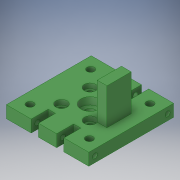
# Autodesk Inventor part: КВ33.044.201 - Щека каретки
Saved by Autodesk Inventor 2019 (Build 230136000, 136)
## iProperties
Created: 2019-07-18
Part Number: КВ33.044.201 - Щека каретки
Material: Пластик АБС
Document SubType Name: Modeling
Designer: Петров Иван
Density: 1.06 g/cm^3
Appearance: Гладкий — темный травянисто-зеленый
Author: Петров Иван
Autodesk Inventor part; units mm, degrees
ref_plane "YZ Plane" through (0, 0, 0) normal (1, 0, 0) x (0, 1, 0)
ref_plane "XZ Plane" through (0, 0, 0) normal (0, 1, 0) x (-1, 0, 0)
ref_plane "XY Plane" through (0, 0, 0) normal (0, 0, 1) x (1, 0, 0)
sketch "Эскиз1" plane through (0, 0, 0) normal (0, 1, 0) x (-1, 0, 0)
  line L0 (-34, 35) -> (34, 35)
  line L1 (34, 35) -> (34, -35)
  line L2 (34, -35) -> (-34, -35)
  line L3 (-34, -35) -> (-34, 35)
  line L4 (-34, 35) -> (34, -35) construction
  line L5 (34, 35) -> (-34, -35) construction
  line L6 (0, -35) -> (0, -25)
  line L7 (0, -25) -> (24.48, -25)
  line L8 (0, -25) -> (-24.48, -25)
  circle A0 centre (24.48, -25) radius 3
  circle A1 centre (-24.48, -25) radius 3
  line L9 (0, 35) -> (0, 25)
  line L10 (0, 25) -> (24.48, 25)
  line L11 (0, 25) -> (24.48, 25) construction
  line L12 (0, 25) -> (-24.48, 25)
  circle A2 centre (-24.48, 25) radius 3
  circle A3 centre (24.48, 25) radius 3
  arc A4 (3.9646, 5.9999) -> (5.0253, 6.4392) centre (3.9646, 7.4999) ccw
  line L13 (3.9646, 5.9999) -> (0.7747, 5.9999)
  line L14 (0.7747, 5.9999) -> (0.0002, 5.35)
  line L15 (0.0002, 5.35) -> (-0.7746, 6.0001)
  line L16 (-0.7746, 6.0001) -> (-3.9642, 6.0001)
  arc A5 (-5.0249, 6.4394) -> (-3.9642, 6.0001) centre (-3.9642, 7.5001) ccw
  line L17 (-5.0249, 6.4394) -> (-8.3536, 9.7681)
  arc A6 (-8.5, 10.1217) -> (-8.3536, 9.7681) centre (-8, 10.1217) ccw
  line L18 (-8.5, 10.1217) -> (-8.5, 12.6)
  arc A7 (-8.3, 12.8) -> (-8.5, 12.6) centre (-8.3, 12.6) ccw
  line L19 (-8.3, 12.8) -> (-4.3, 12.8)
  arc A8 (-4.3, 12.8) -> (-4.1, 13) centre (-4.3, 13) ccw
  line L20 (-4.1, 13) -> (-4.1, 14.1)
  arc A9 (-4.1, 14.1) -> (-4.3, 14.3) centre (-4.3, 14.1) ccw
  line L21 (-4.3, 14.3) -> (-4.7, 14.3)
  line L22 (-4.7, 14.3) -> (-4.7, 14.8001)
  arc A10 (-4.7, 14.8001) -> (-4.9001, 15.0001) centre (-4.9001, 14.8001) ccw
  line L23 (-4.9001, 15.0001) -> (-13.5, 15.0001)
  arc A11 (-13.5, 15.0001) -> (-15, 13.5001) centre (-13.5, 13.5001) ccw
  line L24 (-15, 13.5001) -> (-15, 4.8999)
  arc A12 (-15, 4.8999) -> (-14.8, 4.6999) centre (-14.8, 4.8999) ccw
  line L25 (-14.8, 4.6999) -> (-14.3, 4.6999)
  line L26 (-14.3, 4.6999) -> (-14.3, 4.2999)
  arc A13 (-14.3, 4.2999) -> (-14.1, 4.0999) centre (-14.1, 4.2999) ccw
  line L27 (-14.1, 4.0999) -> (-13, 4.0999)
  arc A14 (-13, 4.0999) -> (-12.8, 4.2999) centre (-13, 4.2999) ccw
  line L28 (-12.8, 4.2999) -> (-12.8, 8.3)
  arc A15 (-12.6, 8.5) -> (-12.8, 8.3) centre (-12.6, 8.3) ccw
  line L29 (-12.6, 8.5) -> (-10.1211, 8.5)
  arc A16 (-9.7675, 8.3536) -> (-10.1211, 8.5) centre (-10.1211, 8) ccw
  line L30 (-9.7675, 8.3536) -> (-6.4392, 5.0253)
  arc A17 (-5.9999, 3.9646) -> (-6.4392, 5.0253) centre (-7.4999, 3.9646) ccw
  line L31 (-5.9999, 3.9646) -> (-5.9999, 0.7747)
  line L32 (-5.9999, 0.7747) -> (-5.35, 0.0002)
  line L33 (-5.35, 0.0002) -> (-6.0001, -0.7746)
  line L34 (-6.0001, -0.7746) -> (-6.0001, -3.9642)
  arc A18 (-6.4394, -5.0249) -> (-6.0001, -3.9642) centre (-7.5001, -3.9642) ccw
  line L35 (-6.4394, -5.0249) -> (-9.7681, -8.3536)
  arc A19 (-10.1217, -8.5) -> (-9.7681, -8.3536) centre (-10.1217, -8) ccw
  line L36 (-10.1217, -8.5) -> (-12.6, -8.5)
  arc A20 (-12.8, -8.3) -> (-12.6, -8.5) centre (-12.6, -8.3) ccw
  line L37 (-12.8, -8.3) -> (-12.8, -4.3)
  arc A21 (-12.8, -4.3) -> (-13, -4.1) centre (-13, -4.3) ccw
  line L38 (-13, -4.1) -> (-14.1, -4.1)
  arc A22 (-14.1, -4.1) -> (-14.3, -4.3) centre (-14.1, -4.3) ccw
  line L39 (-14.3, -4.3) -> (-14.3, -4.7)
  line L40 (-14.3, -4.7) -> (-14.8, -4.7)
  arc A23 (-14.8, -4.7) -> (-15, -4.9) centre (-14.8, -4.9) ccw
  line L41 (-15, -4.9) -> (-15, -13.5)
  arc A24 (-15, -13.5) -> (-13.5, -15) centre (-13.5, -13.5) ccw
  line L42 (-13.5, -15) -> (-4.8998, -15)
  arc A25 (-4.8998, -15) -> (-4.6998, -14.8) centre (-4.8998, -14.8) ccw
  line L43 (-4.6998, -14.8) -> (-4.6998, -14.3)
  line L44 (-4.6998, -14.3) -> (-4.2998, -14.3)
  arc A26 (-4.2998, -14.3) -> (-4.0998, -14.1) centre (-4.2998, -14.1) ccw
  line L45 (-4.0998, -14.1) -> (-4.0998, -13)
  arc A27 (-4.0998, -13) -> (-4.2998, -12.8) centre (-4.2998, -13) ccw
  line L46 (-4.2998, -12.8) -> (-8.2999, -12.8)
  arc A28 (-8.4999, -12.6) -> (-8.2999, -12.8) centre (-8.2999, -12.6) ccw
  line L47 (-8.4999, -12.6) -> (-8.4999, -10.1211)
  arc A29 (-8.3534, -9.7675) -> (-8.4999, -10.1211) centre (-7.9999, -10.1211) ccw
  line L48 (-8.3534, -9.7675) -> (-5.0251, -6.4392)
  arc A30 (-3.9645, -5.9999) -> (-5.0251, -6.4392) centre (-3.9645, -7.4999) ccw
  line L49 (-3.9645, -5.9999) -> (-0.7745, -5.9999)
  line L50 (-0.7745, -5.9999) -> (0, -5.35)
  line L51 (0, -5.35) -> (0.7747, -6.0001)
  line L52 (0.7747, -6.0001) -> (3.9644, -6.0001)
  arc A31 (5.025, -6.4394) -> (3.9644, -6.0001) centre (3.9644, -7.5001) ccw
  line L53 (5.025, -6.4394) -> (8.3537, -9.7681)
  arc A32 (8.5001, -10.1217) -> (8.3537, -9.7681) centre (8.0001, -10.1217) ccw
  line L54 (8.5001, -10.1217) -> (8.5001, -12.6)
  arc A33 (8.3001, -12.8) -> (8.5001, -12.6) centre (8.3001, -12.6) ccw
  line L55 (8.3001, -12.8) -> (4.3002, -12.8)
  arc A34 (4.3002, -12.8) -> (4.1002, -13) centre (4.3002, -13) ccw
  line L56 (4.1002, -13) -> (4.1002, -14.1)
  arc A35 (4.1002, -14.1) -> (4.3002, -14.3) centre (4.3002, -14.1) ccw
  line L57 (4.3002, -14.3) -> (4.7002, -14.3)
  line L58 (4.7002, -14.3) -> (4.7002, -14.8)
  arc A36 (4.7002, -14.8) -> (4.9002, -15) centre (4.9002, -14.8) ccw
  line L59 (4.9002, -15) -> (13.5001, -15)
  arc A37 (13.5001, -15) -> (15.0001, -13.5) centre (13.5001, -13.5) ccw
  line L60 (15.0001, -13.5) -> (15.0001, -4.8998)
  arc A38 (15.0001, -4.8998) -> (14.8001, -4.6998) centre (14.8001, -4.8998) ccw
  line L61 (14.8001, -4.6998) -> (14.3001, -4.6998)
  line L62 (14.3001, -4.6998) -> (14.3001, -4.2998)
  arc A39 (14.3001, -4.2998) -> (14.1001, -4.0998) centre (14.1001, -4.2998) ccw
  line L63 (14.1001, -4.0998) -> (13.0001, -4.0998)
  arc A40 (13.0001, -4.0998) -> (12.8001, -4.2998) centre (13.0001, -4.2998) ccw
  line L64 (12.8001, -4.2998) -> (12.8001, -8.2999)
  arc A41 (12.6001, -8.4999) -> (12.8001, -8.2999) centre (12.6001, -8.2999) ccw
  line L65 (12.6001, -8.4999) -> (10.1212, -8.4999)
  arc A42 (9.7677, -8.3534) -> (10.1212, -8.4999) centre (10.1212, -7.9999) ccw
  line L66 (9.7677, -8.3534) -> (6.4394, -5.0251)
  arc A43 (6, -3.9645) -> (6.4394, -5.0251) centre (7.5, -3.9645) ccw
  line L67 (6, -3.9645) -> (6, -0.7745)
  line L68 (6, -0.7745) -> (5.3501, 0)
  line L69 (5.3501, 0) -> (6.0002, 0.7747)
  line L70 (6.0002, 0.7747) -> (6.0002, 3.9644)
  arc A44 (6.4396, 5.025) -> (6.0002, 3.9644) centre (7.5002, 3.9644) ccw
  line L71 (6.4396, 5.025) -> (9.7682, 8.3537)
  arc A45 (10.1218, 8.5001) -> (9.7682, 8.3537) centre (10.1218, 8.0001) ccw
  line L72 (10.1218, 8.5001) -> (12.6001, 8.5001)
  arc A46 (12.8001, 8.3001) -> (12.6001, 8.5001) centre (12.6001, 8.3001) ccw
  line L73 (12.8001, 8.3001) -> (12.8001, 4.3002)
  arc A47 (12.8001, 4.3002) -> (13.0001, 4.1002) centre (13.0001, 4.3002) ccw
  line L74 (13.0001, 4.1002) -> (14.1001, 4.1002)
  arc A48 (14.1001, 4.1002) -> (14.3001, 4.3002) centre (14.1001, 4.3002) ccw
  line L75 (14.3001, 4.3002) -> (14.3001, 4.7001)
  line L76 (14.3001, 4.7001) -> (14.8001, 4.7001)
  arc A49 (14.8001, 4.7001) -> (15.0001, 4.9001) centre (14.8001, 4.9001) ccw
  line L77 (15.0001, 4.9001) -> (15.0001, 13.5002)
  arc A50 (15.0001, 13.5002) -> (13.5001, 15.0002) centre (13.5001, 13.5002) ccw
  line L78 (13.5001, 15.0002) -> (4.8999, 15.0002)
  arc A51 (4.8999, 15.0002) -> (4.6999, 14.8002) centre (4.8999, 14.8002) ccw
  line L79 (4.6999, 14.8002) -> (4.6999, 14.3)
  line L80 (4.6999, 14.3) -> (4.2999, 14.3)
  arc A52 (4.2999, 14.3) -> (4.0999, 14.1) centre (4.2999, 14.1) ccw
  line L81 (4.0999, 14.1) -> (4.0999, 13)
  arc A53 (4.0999, 13) -> (4.2999, 12.8) centre (4.2999, 13) ccw
  line L82 (4.2999, 12.8) -> (8.3, 12.8)
  arc A54 (8.5, 12.6) -> (8.3, 12.8) centre (8.3, 12.6) ccw
  line L83 (8.5, 12.6) -> (8.5, 10.1211)
  arc A55 (8.3536, 9.7675) -> (8.5, 10.1211) centre (8, 10.1211) ccw
  line L84 (8.3536, 9.7675) -> (5.0253, 6.4392)
  arc A56 (-12.7113, -10.2413) -> (-12.4546, -10.3134) centre (-12.5426, -10.1338) ccw
  arc A57 (-11.0457, -10.3134) -> (-12.4546, -10.3134) centre (-11.7501, -11.75) ccw
  arc A58 (-11.0457, -10.3134) -> (-10.789, -10.2413) centre (-10.9577, -10.1338) ccw
  line L85 (-10.6305, -9.9925) -> (-10.789, -10.2413)
  arc A59 (-10.4618, -9.9) -> (-10.6305, -9.9925) centre (-10.4618, -10.1) ccw
  line L86 (-10.3001, -9.9) -> (-10.4618, -9.9)
  arc A60 (-9.9001, -10.3) -> (-10.3001, -9.9) centre (-10.3001, -10.3) ccw
  line L87 (-9.9001, -10.4617) -> (-9.9001, -10.3)
  arc A61 (-9.9927, -10.6304) -> (-9.9001, -10.4617) centre (-10.1001, -10.4617) ccw
  line L88 (-10.2414, -10.7888) -> (-9.9927, -10.6304)
  arc A62 (-10.2414, -10.7888) -> (-10.3136, -11.0456) centre (-10.134, -10.9575) ccw
  arc A63 (-10.3136, -12.4544) -> (-10.3136, -11.0456) centre (-11.7501, -11.75) ccw
  arc A64 (-10.3136, -12.4544) -> (-10.2414, -12.7111) centre (-10.134, -12.5425) ccw
  line L89 (-9.9927, -12.8696) -> (-10.2414, -12.7111)
  arc A65 (-9.9001, -13.0383) -> (-9.9927, -12.8696) centre (-10.1001, -13.0383) ccw
  line L90 (-9.9001, -13.2) -> (-9.9001, -13.0383)
  arc A66 (-10.3001, -13.6) -> (-9.9001, -13.2) centre (-10.3001, -13.2) ccw
  line L91 (-10.4618, -13.6) -> (-10.3001, -13.6)
  arc A67 (-10.6305, -13.5075) -> (-10.4618, -13.6) centre (-10.4618, -13.4) ccw
  line L92 (-10.789, -13.2587) -> (-10.6305, -13.5075)
  arc A68 (-10.789, -13.2587) -> (-11.0457, -13.1866) centre (-10.9577, -13.3662) ccw
  arc A69 (-12.4546, -13.1866) -> (-11.0457, -13.1866) centre (-11.7501, -11.75) ccw
  arc A70 (-12.4546, -13.1866) -> (-12.7113, -13.2587) centre (-12.5426, -13.3662) ccw
  line L93 (-12.8698, -13.5075) -> (-12.7113, -13.2587)
  arc A71 (-13.0385, -13.6) -> (-12.8698, -13.5075) centre (-13.0385, -13.4) ccw
  line L94 (-13.2001, -13.6) -> (-13.0385, -13.6)
  arc A72 (-13.6001, -13.2) -> (-13.2001, -13.6) centre (-13.2001, -13.2) ccw
  line L95 (-13.6001, -13.0383) -> (-13.6001, -13.2)
  arc A73 (-13.5076, -12.8696) -> (-13.6001, -13.0383) centre (-13.4001, -13.0383) ccw
  line L96 (-13.2589, -12.7111) -> (-13.5076, -12.8696)
  arc A74 (-13.2589, -12.7111) -> (-13.1867, -12.4544) centre (-13.3663, -12.5425) ccw
  arc A75 (-13.1867, -11.0456) -> (-13.1867, -12.4544) centre (-11.7501, -11.75) ccw
  arc A76 (-13.1867, -11.0456) -> (-13.2589, -10.7888) centre (-13.3663, -10.9575) ccw
  line L97 (-13.5076, -10.6304) -> (-13.2589, -10.7888)
  arc A77 (-13.6001, -10.4617) -> (-13.5076, -10.6304) centre (-13.4001, -10.4617) ccw
  line L98 (-13.6001, -10.3) -> (-13.6001, -10.4617)
  arc A78 (-13.2001, -9.9) -> (-13.6001, -10.3) centre (-13.2001, -10.3) ccw
  line L99 (-13.0385, -9.9) -> (-13.2001, -9.9)
  arc A79 (-12.8698, -9.9925) -> (-13.0385, -9.9) centre (-13.0385, -10.1) ccw
  line L100 (-12.7113, -10.2413) -> (-12.8698, -9.9925)
  arc A80 (10.2413, -12.7113) -> (10.3134, -12.4546) centre (10.1338, -12.5426) ccw
  arc A81 (10.3134, -11.0457) -> (10.3134, -12.4546) centre (11.75, -11.7501) ccw
  arc A82 (10.3134, -11.0457) -> (10.2413, -10.789) centre (10.1338, -10.9577) ccw
  line L101 (9.9925, -10.6305) -> (10.2413, -10.789)
  arc A83 (9.9, -10.4618) -> (9.9925, -10.6305) centre (10.1, -10.4618) ccw
  line L102 (9.9, -10.3001) -> (9.9, -10.4618)
  arc A84 (10.3, -9.9001) -> (9.9, -10.3001) centre (10.3, -10.3001) ccw
  line L103 (10.4617, -9.9001) -> (10.3, -9.9001)
  arc A85 (10.6304, -9.9927) -> (10.4617, -9.9001) centre (10.4617, -10.1001) ccw
  line L104 (10.7888, -10.2414) -> (10.6304, -9.9927)
  arc A86 (10.7888, -10.2414) -> (11.0456, -10.3136) centre (10.9575, -10.134) ccw
  arc A87 (12.4544, -10.3136) -> (11.0456, -10.3136) centre (11.75, -11.7501) ccw
  arc A88 (12.4544, -10.3136) -> (12.7111, -10.2414) centre (12.5425, -10.134) ccw
  line L105 (12.8696, -9.9927) -> (12.7111, -10.2414)
  arc A89 (13.0383, -9.9001) -> (12.8696, -9.9927) centre (13.0383, -10.1001) ccw
  line L106 (13.2, -9.9001) -> (13.0383, -9.9001)
  arc A90 (13.6, -10.3001) -> (13.2, -9.9001) centre (13.2, -10.3001) ccw
  line L107 (13.6, -10.4618) -> (13.6, -10.3001)
  arc A91 (13.5075, -10.6305) -> (13.6, -10.4618) centre (13.4, -10.4618) ccw
  line L108 (13.2587, -10.789) -> (13.5075, -10.6305)
  arc A92 (13.2587, -10.789) -> (13.1866, -11.0457) centre (13.3662, -10.9577) ccw
  arc A93 (13.1866, -12.4546) -> (13.1866, -11.0457) centre (11.75, -11.7501) ccw
  arc A94 (13.1866, -12.4546) -> (13.2587, -12.7113) centre (13.3662, -12.5426) ccw
  line L109 (13.5075, -12.8698) -> (13.2587, -12.7113)
  arc A95 (13.6, -13.0385) -> (13.5075, -12.8698) centre (13.4, -13.0385) ccw
  line L110 (13.6, -13.2001) -> (13.6, -13.0385)
  arc A96 (13.2, -13.6001) -> (13.6, -13.2001) centre (13.2, -13.2001) ccw
  line L111 (13.0383, -13.6001) -> (13.2, -13.6001)
  arc A97 (12.8696, -13.5076) -> (13.0383, -13.6001) centre (13.0383, -13.4001) ccw
  line L112 (12.7111, -13.2589) -> (12.8696, -13.5076)
  arc A98 (12.7111, -13.2589) -> (12.4544, -13.1867) centre (12.5425, -13.3663) ccw
  arc A99 (11.0456, -13.1867) -> (12.4544, -13.1867) centre (11.75, -11.7501) ccw
  arc A100 (11.0456, -13.1867) -> (10.7888, -13.2589) centre (10.9575, -13.3663) ccw
  line L113 (10.6304, -13.5076) -> (10.7888, -13.2589)
  arc A101 (10.4617, -13.6001) -> (10.6304, -13.5076) centre (10.4617, -13.4001) ccw
  line L114 (10.3, -13.6001) -> (10.4617, -13.6001)
  arc A102 (9.9, -13.2001) -> (10.3, -13.6001) centre (10.3, -13.2001) ccw
  line L115 (9.9, -13.0385) -> (9.9, -13.2001)
  arc A103 (9.9925, -12.8698) -> (9.9, -13.0385) centre (10.1, -13.0385) ccw
  line L116 (10.2413, -12.7113) -> (9.9925, -12.8698)
  arc A104 (3.1213, -1.5836) -> (3.1996, -1.8473) centre (3.2996, -1.6741) ccw
  line L117 (3.7642, -2.1733) -> (3.1996, -1.8473)
  arc A105 (3.7642, -2.1733) -> (4.0056, -2.1415) centre (3.8642, -2.0001) ccw
  line L118 (4.1586, -1.9885) -> (4.0056, -2.1415)
  arc A106 (4.5, -2.13) -> (4.1586, -1.9885) centre (4.3, -2.13) ccw
  line L119 (4.5, -3.5) -> (4.5, -2.13)
  arc A107 (3.5, -4.5) -> (4.5, -3.5) centre (3.5, -3.5) ccw
  line L120 (2.13, -4.5) -> (3.5, -4.5)
  arc A108 (1.9885, -4.1586) -> (2.13, -4.5) centre (2.13, -4.3) ccw
  line L121 (2.1415, -4.0056) -> (1.9885, -4.1586)
  arc A109 (2.1415, -4.0056) -> (2.1733, -3.7642) centre (2.0001, -3.8642) ccw
  line L122 (1.8473, -3.1996) -> (2.1733, -3.7642)
  arc A110 (1.8473, -3.1996) -> (1.5836, -3.1213) centre (1.6741, -3.2996) ccw
  arc A111 (-1.5836, -3.1213) -> (1.5836, -3.1213) centre (0, 0) ccw
  arc A112 (-1.5836, -3.1213) -> (-1.8473, -3.1996) centre (-1.6741, -3.2996) ccw
  line L123 (-2.1733, -3.7642) -> (-1.8473, -3.1996)
  arc A113 (-2.1733, -3.7642) -> (-2.1415, -4.0056) centre (-2.0001, -3.8642) ccw
  line L124 (-1.9885, -4.1586) -> (-2.1415, -4.0056)
  arc A114 (-2.13, -4.5) -> (-1.9885, -4.1586) centre (-2.13, -4.3) ccw
  line L125 (-3.5, -4.5) -> (-2.13, -4.5)
  arc A115 (-4.5, -3.5) -> (-3.5, -4.5) centre (-3.5, -3.5) ccw
  line L126 (-4.5, -2.13) -> (-4.5, -3.5)
  arc A116 (-4.1586, -1.9885) -> (-4.5, -2.13) centre (-4.3, -2.13) ccw
  line L127 (-4.0056, -2.1415) -> (-4.1586, -1.9885)
  arc A117 (-4.0056, -2.1415) -> (-3.7642, -2.1733) centre (-3.8642, -2.0001) ccw
  line L128 (-3.1996, -1.8473) -> (-3.7642, -2.1733)
  arc A118 (-3.1996, -1.8473) -> (-3.1213, -1.5836) centre (-3.2996, -1.6741) ccw
  arc A119 (-3.1213, 1.5836) -> (-3.1213, -1.5836) centre (0, 0) ccw
  arc A120 (-3.1213, 1.5836) -> (-3.1996, 1.8473) centre (-3.2996, 1.6741) ccw
  line L129 (-3.7642, 2.1733) -> (-3.1996, 1.8473)
  arc A121 (-3.7642, 2.1733) -> (-4.0056, 2.1415) centre (-3.8642, 2.0001) ccw
  line L130 (-4.1586, 1.9885) -> (-4.0056, 2.1415)
  arc A122 (-4.5, 2.13) -> (-4.1586, 1.9885) centre (-4.3, 2.13) ccw
  line L131 (-4.5, 3.5) -> (-4.5, 2.13)
  arc A123 (-3.5, 4.5) -> (-4.5, 3.5) centre (-3.5, 3.5) ccw
  line L132 (-2.13, 4.5) -> (-3.5, 4.5)
  arc A124 (-1.9885, 4.1586) -> (-2.13, 4.5) centre (-2.13, 4.3) ccw
  line L133 (-2.1415, 4.0056) -> (-1.9885, 4.1586)
  arc A125 (-2.1415, 4.0056) -> (-2.1733, 3.7642) centre (-2.0001, 3.8642) ccw
  line L134 (-1.8473, 3.1996) -> (-2.1733, 3.7642)
  arc A126 (-1.8473, 3.1996) -> (-1.5836, 3.1213) centre (-1.6741, 3.2996) ccw
  arc A127 (1.5836, 3.1213) -> (-1.5836, 3.1213) centre (0, 0) ccw
  arc A128 (1.5836, 3.1213) -> (1.8473, 3.1996) centre (1.6741, 3.2996) ccw
  line L135 (2.1733, 3.7642) -> (1.8473, 3.1996)
  arc A129 (2.1733, 3.7642) -> (2.1415, 4.0056) centre (2.0001, 3.8642) ccw
  line L136 (1.9885, 4.1586) -> (2.1415, 4.0056)
  arc A130 (2.13, 4.5) -> (1.9885, 4.1586) centre (2.13, 4.3) ccw
  line L137 (3.5, 4.5) -> (2.13, 4.5)
  arc A131 (4.5, 3.5) -> (3.5, 4.5) centre (3.5, 3.5) ccw
  line L138 (4.5, 2.13) -> (4.5, 3.5)
  arc A132 (4.1586, 1.9885) -> (4.5, 2.13) centre (4.3, 2.13) ccw
  line L139 (4.0056, 2.1415) -> (4.1586, 1.9885)
  arc A133 (4.0056, 2.1415) -> (3.7642, 2.1733) centre (3.8642, 2.0001) ccw
  line L140 (3.1996, 1.8473) -> (3.7642, 2.1733)
  arc A134 (3.1996, 1.8473) -> (3.1213, 1.5836) centre (3.2996, 1.6741) ccw
  arc A135 (3.1213, -1.5836) -> (3.1213, 1.5836) centre (0, 0) ccw
  arc A136 (12.7113, 10.2413) -> (12.4546, 10.3134) centre (12.5426, 10.1338) ccw
  arc A137 (11.0457, 10.3134) -> (12.4546, 10.3134) centre (11.7501, 11.75) ccw
  arc A138 (11.0457, 10.3134) -> (10.789, 10.2413) centre (10.9577, 10.1338) ccw
  line L141 (10.6305, 9.9925) -> (10.789, 10.2413)
  arc A139 (10.4618, 9.9) -> (10.6305, 9.9925) centre (10.4618, 10.1) ccw
  line L142 (10.3001, 9.9) -> (10.4618, 9.9)
  arc A140 (9.9001, 10.3) -> (10.3001, 9.9) centre (10.3001, 10.3) ccw
  line L143 (9.9001, 10.4617) -> (9.9001, 10.3)
  arc A141 (9.9927, 10.6304) -> (9.9001, 10.4617) centre (10.1001, 10.4617) ccw
  line L144 (10.2414, 10.7888) -> (9.9927, 10.6304)
  arc A142 (10.2414, 10.7888) -> (10.3136, 11.0456) centre (10.134, 10.9575) ccw
  arc A143 (10.3136, 12.4544) -> (10.3136, 11.0456) centre (11.7501, 11.75) ccw
  arc A144 (10.3136, 12.4544) -> (10.2414, 12.7111) centre (10.134, 12.5425) ccw
  line L145 (9.9927, 12.8696) -> (10.2414, 12.7111)
  arc A145 (9.9001, 13.0383) -> (9.9927, 12.8696) centre (10.1001, 13.0383) ccw
  line L146 (9.9001, 13.2) -> (9.9001, 13.0383)
  arc A146 (10.3001, 13.6) -> (9.9001, 13.2) centre (10.3001, 13.2) ccw
  line L147 (10.4618, 13.6) -> (10.3001, 13.6)
  arc A147 (10.6305, 13.5075) -> (10.4618, 13.6) centre (10.4618, 13.4) ccw
  line L148 (10.789, 13.2587) -> (10.6305, 13.5075)
  arc A148 (10.789, 13.2587) -> (11.0457, 13.1866) centre (10.9577, 13.3662) ccw
  arc A149 (12.4546, 13.1866) -> (11.0457, 13.1866) centre (11.7501, 11.75) ccw
  arc A150 (12.4546, 13.1866) -> (12.7113, 13.2587) centre (12.5426, 13.3662) ccw
  line L149 (12.8698, 13.5075) -> (12.7113, 13.2587)
  arc A151 (13.0385, 13.6) -> (12.8698, 13.5075) centre (13.0385, 13.4) ccw
  line L150 (13.2001, 13.6) -> (13.0385, 13.6)
  arc A152 (13.6001, 13.2) -> (13.2001, 13.6) centre (13.2001, 13.2) ccw
  line L151 (13.6001, 13.0383) -> (13.6001, 13.2)
  arc A153 (13.5076, 12.8696) -> (13.6001, 13.0383) centre (13.4001, 13.0383) ccw
  line L152 (13.2589, 12.7111) -> (13.5076, 12.8696)
  arc A154 (13.2589, 12.7111) -> (13.1867, 12.4544) centre (13.3663, 12.5425) ccw
  arc A155 (13.1867, 11.0456) -> (13.1867, 12.4544) centre (11.7501, 11.75) ccw
  arc A156 (13.1867, 11.0456) -> (13.2589, 10.7888) centre (13.3663, 10.9575) ccw
  line L153 (13.5076, 10.6304) -> (13.2589, 10.7888)
  arc A157 (13.6001, 10.4617) -> (13.5076, 10.6304) centre (13.4001, 10.4617) ccw
  line L154 (13.6001, 10.3) -> (13.6001, 10.4617)
  arc A158 (13.2001, 9.9) -> (13.6001, 10.3) centre (13.2001, 10.3) ccw
  line L155 (13.0385, 9.9) -> (13.2001, 9.9)
  arc A159 (12.8698, 9.9925) -> (13.0385, 9.9) centre (13.0385, 10.1) ccw
  line L156 (12.7113, 10.2413) -> (12.8698, 9.9925)
  arc A160 (-10.2413, 12.7113) -> (-10.3134, 12.4546) centre (-10.1338, 12.5426) ccw
  arc A161 (-10.3134, 11.0457) -> (-10.3134, 12.4546) centre (-11.75, 11.7501) ccw
  arc A162 (-10.3134, 11.0457) -> (-10.2413, 10.789) centre (-10.1338, 10.9577) ccw
  line L157 (-9.9925, 10.6305) -> (-10.2413, 10.789)
  arc A163 (-9.9, 10.4618) -> (-9.9925, 10.6305) centre (-10.1, 10.4618) ccw
  line L158 (-9.9, 10.3001) -> (-9.9, 10.4618)
  arc A164 (-10.3, 9.9001) -> (-9.9, 10.3001) centre (-10.3, 10.3001) ccw
  line L159 (-10.4617, 9.9001) -> (-10.3, 9.9001)
  arc A165 (-10.6304, 9.9927) -> (-10.4617, 9.9001) centre (-10.4617, 10.1001) ccw
  line L160 (-10.7888, 10.2414) -> (-10.6304, 9.9927)
  arc A166 (-10.7888, 10.2414) -> (-11.0456, 10.3136) centre (-10.9575, 10.134) ccw
  arc A167 (-12.4544, 10.3136) -> (-11.0456, 10.3136) centre (-11.75, 11.7501) ccw
  arc A168 (-12.4544, 10.3136) -> (-12.7111, 10.2414) centre (-12.5425, 10.134) ccw
  line L161 (-12.8696, 9.9927) -> (-12.7111, 10.2414)
  arc A169 (-13.0383, 9.9001) -> (-12.8696, 9.9927) centre (-13.0383, 10.1001) ccw
  line L162 (-13.2, 9.9001) -> (-13.0383, 9.9001)
  arc A170 (-13.6, 10.3001) -> (-13.2, 9.9001) centre (-13.2, 10.3001) ccw
  line L163 (-13.6, 10.4618) -> (-13.6, 10.3001)
  arc A171 (-13.5075, 10.6305) -> (-13.6, 10.4618) centre (-13.4, 10.4618) ccw
  line L164 (-13.2587, 10.789) -> (-13.5075, 10.6305)
  arc A172 (-13.2587, 10.789) -> (-13.1866, 11.0457) centre (-13.3662, 10.9577) ccw
  arc A173 (-13.1866, 12.4546) -> (-13.1866, 11.0457) centre (-11.75, 11.7501) ccw
  arc A174 (-13.1866, 12.4546) -> (-13.2587, 12.7113) centre (-13.3662, 12.5426) ccw
  line L165 (-13.5075, 12.8698) -> (-13.2587, 12.7113)
  arc A175 (-13.6, 13.0385) -> (-13.5075, 12.8698) centre (-13.4, 13.0385) ccw
  line L166 (-13.6, 13.2001) -> (-13.6, 13.0385)
  arc A176 (-13.2, 13.6001) -> (-13.6, 13.2001) centre (-13.2, 13.2001) ccw
  line L167 (-13.0383, 13.6001) -> (-13.2, 13.6001)
  arc A177 (-12.8696, 13.5076) -> (-13.0383, 13.6001) centre (-13.0383, 13.4001) ccw
  line L168 (-12.7111, 13.2589) -> (-12.8696, 13.5076)
  arc A178 (-12.7111, 13.2589) -> (-12.4544, 13.1867) centre (-12.5425, 13.3663) ccw
  arc A179 (-11.0456, 13.1867) -> (-12.4544, 13.1867) centre (-11.75, 11.7501) ccw
  arc A180 (-11.0456, 13.1867) -> (-10.7888, 13.2589) centre (-10.9575, 13.3663) ccw
  line L169 (-10.6304, 13.5076) -> (-10.7888, 13.2589)
  arc A181 (-10.4617, 13.6001) -> (-10.6304, 13.5076) centre (-10.4617, 13.4001) ccw
  line L170 (-10.3, 13.6001) -> (-10.4617, 13.6001)
  arc A182 (-9.9, 13.2001) -> (-10.3, 13.6001) centre (-10.3, 13.2001) ccw
  line L171 (-9.9, 13.0385) -> (-9.9, 13.2001)
  arc A183 (-9.9925, 12.8698) -> (-9.9, 13.0385) centre (-10.1, 13.0385) ccw
  line L172 (-10.2413, 12.7113) -> (-9.9925, 12.8698)
  circle A184 centre (0, 0) radius 4.1
  circle A185 centre (-11.75, 11.7501) radius 1.6
  circle A186 centre (11.7501, 11.75) radius 1.6
  circle A187 centre (11.75, -11.7501) radius 1.6
  circle A188 centre (-11.7501, -11.75) radius 1.6
  dimension "d46" = 3.2
  dimension "d0" = 68
  dimension "d1" = 70
  dimension "d2" = 10
  dimension "d3" = 24.48
  dimension "d4" = 24.48
  dimension "d5" = 6
  dimension "d6" = 6
  dimension "d7" = 10
  dimension "d8" = 24.48
  dimension "d9" = 0
  dimension "d10" = 24.48
  dimension "d11" = 6
  dimension "d12" = 6
  dimension "d33" = 8.2
  constraints: 360 point on circle, 346 end point, 188 centre point, 8 coincident, 5 horizontal, 2 midpoint, 2 parallel, 2 perpendicular, 2 vertical, 1 collinear, 3 other
  measures "d0" distance of L1.end L2.end
  measures "d1" distance of L0.end L1.end
  measures "d2" distance of L6.start L6.end
  measures "d3" distance of L6.end L7.end
  measures "d4" distance of L6.end L8.end
  measures "d5" diameter of A0
  measures "d6" diameter of A1
  measures "d7" distance of L9.start L9.end
  measures "d8" distance of L9.end L10.end
  measures "d9" distance between parallel lines of L10 L11
  measures "d10" distance of L9.end L12.end
  measures "d11" diameter of A2
  measures "d12" diameter of A3
  measures "d33" diameter of A184
extrude "Выдавливание1" add sketch "Эскиз1" along normal blind 10 contours L0 L1 L2 L3 | A4 L84 A55 L83 A54 L82 A53 L81 A52 L80 L79 A51 L78 A50 L77 A49 L76 L75 A48 L74 A47 L73 A46 L72 A45 L71 A44 L70 L69 L68 L67 A43 L66 A42 L65 A41 L64 A40 L63 A39 L62 L61 A38 L60 A37 L59 A36 L58 L57 A35 L56 A34 L55 A33 L54 A32 L53 A31 L52 L51 L50 L49 A30 L48 A29 L47 A28 L46 A27 L45 A26 L44 L43 A25 L42 A24 L41 A23 L40 L39 A22 L38 A21 L37 A20 L36 A19 L35 A18 L34 L33 L32 L31 A17 L30 A16 L29 A15 L28 A14 L27 A13 L26 L25 A12 L24 A11 L23 A10 L22 L21 A9 L20 A8 L19 A7 L18 A6 L17 A5 L16 L15 L14 L13 | A56 A188 A76 L97 A77 L98 A78 L99 A79 L100 | A58 L85 A59 L86 A60 L87 A61 L88 A62 A188 | A188 A70 L93 A71 L94 A72 L95 A73 L96 A74 | A64 L89 A65 L90 A66 L91 A67 L92 A68 A188 | A80 A187 A100 L113 A101 L114 A102 L115 A103 L116 | A82 L101 A83 L102 A84 L103 A85 L104 A86 A187 | A187 A94 L109 A95 L110 A96 L111 A97 L112 A98 | A88 L105 A89 L106 A90 L107 A91 L108 A92 A187 | L117 A105 L118 A106 L119 A107 L120 A108 L121 A109 L122 A184 | A184 L135 A129 L136 A130 L137 A131 L138 A132 L139 A133 L140 | L123 A113 L124 A114 L125 A115 L126 A116 L127 A117 L128 A184 | A184 L129 A121 L130 A122 L131 A123 L132 A124 L133 A125 L134 | A136 A186 A156 L153 A157 L154 A158 L155 A159 L156 | A138 L141 A139 L142 A140 L143 A141 L144 A142 A186 | A144 L145 A145 L146 A146 L147 A147 L148 A148 A186 | A186 A150 L149 A151 L150 A152 L151 A153 L152 A154 | A160 A185 A180 L169 A181 L170 A182 L171 A183 L172 | A162 L157 A163 L158 A164 L159 A165 L160 A166 A185 | A185 A174 L165 A175 L166 A176 L167 A177 L168 A178 | A168 L161 A169 L162 A170 L163 A171 L164 A172 A185
sketch "Эскиз2" plane through (0, 10, 0) normal (0, 1, 0) x (1, 0, 0)
  line L0 (34, 35) -> (-34, 35) projected
  line L1 (-13.5, 35) -> (-7.5, 35)
  line L2 (-7.5, 35) -> (-7.5, 21)
  line L3 (-7.5, 21) -> (-13.5, 21)
  line L4 (-13.5, 21) -> (-13.5, 35)
  line L5 (34, 35) -> (-34, 35) projected
  line L6 (7.5, 35) -> (13.5, 35)
  line L7 (13.5, 35) -> (13.5, 21)
  line L8 (13.5, 21) -> (7.5, 21)
  line L9 (7.5, 21) -> (7.5, 35)
  line L10 (-34, -35) -> (34, -35) projected
  line L11 (-13.5, -35) -> (-7.5, -35)
  line L12 (-7.5, -35) -> (-7.5, -21)
  line L13 (-7.5, -21) -> (-13.5, -21)
  line L14 (-13.5, -21) -> (-13.5, -35)
  line L15 (7.5, -21) -> (13.5, -21)
  line L16 (13.5, -21) -> (13.5, -35)
  line L17 (13.5, -35) -> (7.5, -35)
  line L18 (7.5, -35) -> (7.5, -21)
  dimension "d53" = 14
  dimension "d54" = 14
  dimension "d55" = 14
  dimension "d56" = 6
  dimension "d57" = 14
  dimension "d58" = 6
  dimension "d59" = 6
  dimension "d60" = 6
  constraints: 32 end point, 8 parallel, 4 horizontal, 4 perpendicular, 4 point on line
  measures "d53" distance of L1.end L2.end
  measures "d54" distance of L6.end L7.end
  measures "d55" distance of L12.end L11.end
  measures "d56" distance of L16.end L17.end
  measures "d57" distance of L15.end L16.end
  measures "d58" distance of L2.end L3.end
  measures "d59" distance of L7.end L8.end
  measures "d60" distance of L11.start L11.end
extrude "Выдавливание2" cut sketch "Эскиз2" against normal blind 10
sketch "Эскиз6" plane through (0, 10, 0) normal (0, 1, 0) x (1, 0, 0)
  circle A0 centre (0, 0) radius 7.5
  dimension "d37" = 15
  constraints: 1 centre point, 1 coincident
  measures "d37" diameter of A0
extrude "Выдавливание6" cut sketch "Эскиз6" against normal blind 6
sketch "Эскиз7" plane through (0, 10, 0) normal (0, 1, 0) x (1, 0, 0)
  circle A0 centre (-11.7501, -11.75) radius 1.6 projected
  circle A1 centre (-11.7501, -11.75) radius 4.65
  circle A2 centre (-11.75, 11.7501) radius 1.6 projected
  circle A3 centre (-11.75, 11.7501) radius 4.65
  circle A4 centre (11.7501, 11.75) radius 1.6 projected
  circle A5 centre (11.7501, 11.75) radius 4.65
  circle A6 centre (11.75, -11.7501) radius 1.6 projected
  circle A7 centre (11.75, -11.7501) radius 4.65
  point P0 (0, 0)
  dimension "d40" = 9.3
  dimension "d41" = 9.3
  dimension "d42" = 9.3
  dimension "d43" = 9.3
  constraints: 4 centre point, 4 coincident
  measures "d40" diameter of A1
  measures "d41" diameter of A3
  measures "d42" diameter of A5
  measures "d43" diameter of A7
extrude "Выдавливание7" cut sketch "Эскиз7" against normal blind 4
sketch "Эскиз8" plane through (-11.7501, 6, 11.75) normal (0, 1, 0) x (1, 0, 0)
  circle A0 centre (0, 0) radius 2.6
  circle A1 centre (0.0001, 23.5001) radius 1.6 projected
  circle A2 centre (0.0001, 23.5001) radius 2.6
  circle A3 centre (23.5003, 23.5) radius 1.6 projected
  circle A4 centre (23.5003, 23.5) radius 2.6
  circle A5 centre (23.5001, -0.0001) radius 1.6 projected
  circle A6 centre (23.5001, -0.0001) radius 2.6
  point P0 (11.7501, 11.75)
  dimension "d47" = 5.2
  dimension "d48" = 5.2
  dimension "d49" = 5.2
  dimension "d50" = 5.2
  constraints: 4 centre point, 3 coincident
  measures "d47" diameter of A0
  measures "d48" diameter of A2
  measures "d49" diameter of A4
  measures "d50" diameter of A6
extrude "Выдавливание8" cut sketch "Эскиз8" against normal blind 10 contours A0 | A1 | A2 | A3 | A4 | A5 | A6
sketch "Эскиз9" plane through (34, 0, 35) normal (1, 0, 0) x (0, 0, -1)
  line L0 (0, 10) -> (0, 0) projected
  line L1 (0, 5) -> (5, 5)
  circle A0 centre (5, 5) radius 2.1
  line L2 (70, 0) -> (70, 10) projected
  line L3 (70, 5) -> (65, 5)
  circle A1 centre (65, 5) radius 2.1
  point P0 (35, 0)
  dimension "d61" = 5
  dimension "d62" = 4.2
  dimension "d65" = 5
  dimension "d66" = 4.2
  constraints: 4 end point, 2 centre point, 2 coincident, 2 horizontal, 2 midpoint
  measures "d61" distance of L1.start L1.end
  measures "d62" diameter of A0
  measures "d65" distance of L3.start L3.end
  measures "d66" diameter of A1
extrude "Выдавливание9" cut sketch "Эскиз9" against normal blind 70
sketch "Эскиз10" plane through (0, 10, 0) normal (0, 1, 0) x (1, 0, 0)
  line L0 (16, -10) -> (24, -10)
  line L1 (24, -10) -> (24, 10)
  line L2 (24, 10) -> (16, 10)
  line L3 (16, 10) -> (16, -10)
  line L4 (16, -10) -> (24, 10) construction
  line L5 (24, -10) -> (16, 10) construction
  line L6 (34, -35) -> (34, 35) projected
  point P0 (0, 0)
  point P1 (20, 0)
  dimension "d67" = 8
  dimension "d68" = 20
  dimension "d71" = 10
  constraints: 12 end point, 2 midpoint, 2 parallel, 1 horizontal, 1 perpendicular
  measures "d67" distance of L2.end L1.end
  measures "d68" distance of L1.end L0.end
  measures "d71" distance between parallel lines of L6 L1
extrude "Выдавливание10" add sketch "Эскиз10" along normal blind 30
equation "\"d4\" = d3"
equation "\"d6\" = d5"
equation "\"d7\" = d2"
equation "\"d8\" = d3"
equation "\"d10\" = d3"
equation "\"d11\" = d5"
equation "\"d12\" = d5"
equation "\"d54\" = d53"
equation "\"d55\" = d53"
equation "\"d56\" = d58"
equation "\"d57\" = d53"
equation "\"d59\" = d58"
equation "\"d60\" = d58"
equation "\"d40\" = d41"
equation "\"d42\" = d41"
equation "\"d43\" = d41"
equation "\"d65\" = d61"
equation "\"d66\" = d62"
